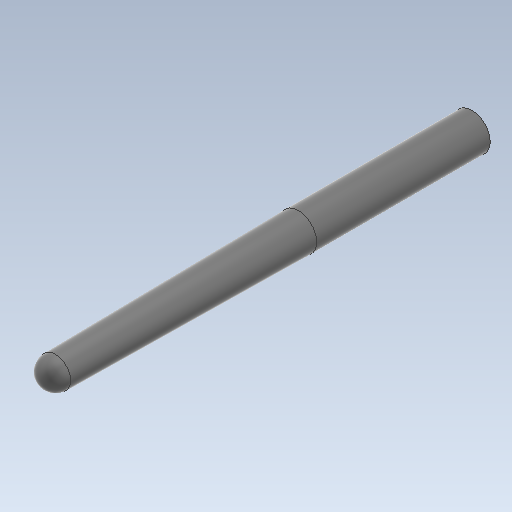
# Autodesk Inventor part: Antenna
Saved by Autodesk Inventor 2020 (Build 240168000, 168)
## iProperties
Created: 2021-06-10
Part Number: Antenna
Material: アセタール樹脂、黒
Document SubType Name: Modeling
Designer: Masato Kubotera
Density: 1.425 g/cm^3
Appearance: 滑らか - 黒
Mass: 10.1482 g
Surface Area: 32.4643 cm^2
Volume: 7.12157 cm^3
Author: Masato Kubotera
Title: Antenna
Autodesk Inventor part; units mm, degrees
ref_plane "YZ Plane" through (0, 0, 0) normal (1, 0, 0) x (0, 1, 0)
ref_plane "XZ Plane" through (0, 0, 0) normal (0, 1, 0) x (-1, 0, 0)
ref_plane "XY Plane" through (0, 0, 0) normal (0, 0, 1) x (1, 0, 0)
sketch "スケッチ2" plane through (0, 0, 0) normal (0, 1, 0) x (-1, 0, 0)
  line L0 (0, 0) -> (-4.75, 0)
  line L1 (0, 112) -> (0, 0)
  line L2 (-4.75, 0) -> (-4.75, 45)
  arc A0 (0, 112) -> (-3.9997, 108.0476) centre (0, 108) ccw
  line L3 (-4.75, 45) -> (-3.9997, 108.0476)
  dimension "d4" = 4.75
  dimension "d6" = 112
  dimension "d8" = 45
  dimension "d9" = 4
  constraints: 8 end point, 2 point on circle, 1 centre point, 1 horizontal, 1 perpendicular, 1 point on line, 1 tangent, 1 vertical
  measures "d4" distance of L0.start L0.end
  measures "d6" distance of L0.start L1.start
  measures "d8" distance of L0.end L2.end
  measures "d9" radius of A0
revolve "回転1" add sketch "スケッチ2" angle 360 about axis through (0, 0, 112) along (0, 0, -1)
